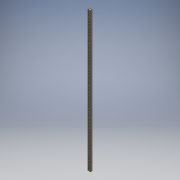
# Autodesk Inventor part: Couvre-Radiateur
Saved by Autodesk Inventor 2016 SP1 (Build 200210100, 210)
## iProperties
Created: 2016-10-06
Part Number: Couvre-Radiateur
Material: Bois (Chêne)
Document SubType Name: Modeling
Designer: dimercur
Density: 0.76 g/cm^3
Appearance: Contreplaqué - Altéré
Mass: 292440 g
Surface Area: 89074 cm^2
Volume: 384790 cm^3
Author: dimercur
Autodesk Inventor part; units mm, degrees
ref_plane "YZ Plane" through (0, 0, 0) normal (1, 0, 0) x (0, 1, 0)
ref_plane "XZ Plane" through (0, 0, 0) normal (0, 1, 0) x (-1, 0, 0)
ref_plane "XY Plane" through (0, 0, 0) normal (0, 0, 1) x (1, 0, 0)
sketch "Esquisse1" plane through (0, 0, 0) normal (0, 1, 0) x (-1, 0, 0)
  line L0 (115, 5975) -> (-115, 5975)
  line L1 (-115, 5975) -> (-115, -5975)
  line L2 (-115, -5975) -> (115, -5975)
  line L3 (115, -5975) -> (115, 5975)
  point P0 (0, 0)
  dimension "d0" = 11950
  dimension "d1" = 230
  dimension "d2" = 115
  dimension "d3" = 5975
  constraints: 8 end point, 2 parallel, 1 horizontal, 1 perpendicular
  measures "d0" distance of L2.end L0.start
  measures "d1" distance of L0.start L0.end
  measures "d2" horizontal distance of point (0, 0) L0.start
  measures "d3" vertical distance of point (0, 0) L0.start
extrude "Extrusion1" add sketch "Esquisse1" along normal blind 140
sketch "Esquisse2" plane through (0, 140, 0) normal (0, 1, 0) x (1, 0, 0)
  line L0 (-65, -5955) -> (65, -5955)
  line L1 (65, -5955) -> (65, -5920)
  line L2 (65, -5920) -> (-65, -5920)
  line L3 (-65, -5920) -> (-65, -5955)
  line L4 (-115, -5975) -> (115, -5975) projected
  line L5 (115, -5975) -> (115, 5975) projected
  point P0 (0, 0)
  dimension "d6" = 35
  dimension "d7" = 130
  dimension "d8" = 20
  dimension "d9" = 50
  constraints: 8 end point, 2 parallel, 1 horizontal, 1 perpendicular
  measures "d6" distance of L2.end L0.start
  measures "d7" distance of L0.start L0.end
  measures "d8" distance from line of L4 L0.start
  measures "d9" distance between parallel lines of L5 L1
extrude "Extrusion2" cut sketch "Esquisse2" against normal through all
pattern_linear "Réseau rectangulaire1" count 216 spacing 55 along (0, 0, -1) of "Extrusion2"
equation "\"d2\" = 0.5 * d1"
equation "\"d3\" = 0.5 * d0"
